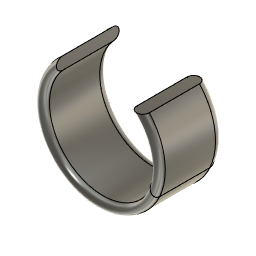
Correa (Autodesk Fusion 360 design; units mm, degrees)
Autodesk Fusion 360 part; units mm, degrees
sketch "Boceto1" plane through (0, 0, 0) normal (0, 0, 1) x (1, 0, 0)
  line L0 (0, 0) -> (30, 0)
  line L1 (30, 0) -> (30, 57)
  line L2 (30, 57) -> (0, 57)
  line L3 (0, 57) -> (0, 0)
  dimension "d1" = 57
  dimension "d2" = 30
  constraint horizontal L0
  constraint vertical L1
  constraint horizontal L2
  constraint vertical L3
  constraint coincident L0.start L3.end
  measures "d1" distance of L0.end L1.end
  measures "d2" distance of L1.end L2.end
extrude "Extruir1" add sketch "Boceto1" along normal blind 3 makes body 1
sketch "Boceto2" plane through (0, 0, 0) normal (0, 0, -1) x (1, 0, 0)
  line L0 (0, 0) -> (0, -57)
  line L1 (0, -57) -> (30, -57)
  line L2 (30, -57) -> (30, 0)
  line L3 (30, 0) -> (0, 0)
extrude "Extruir2" add sketch "Boceto2" against normal blind 10 thin wall 1 outside bodies 1
sketch "Boceto3" plane through (0, 58, 0) normal (0, 1, 0) x (-1, 0, 0)
  line L0 (-31, 0) -> (1, 0)
  line L1 (1, 0) -> (1, 10)
  line L2 (1, 10) -> (-31, 10)
  line L3 (-31, 10) -> (-31, 0)
  line L4 (-22.5, 6.5) -> (-7.5, 6.5)
  line L5 (-7.5, 6.5) -> (-7.5, 3.5)
  line L6 (-7.5, 3.5) -> (-22.5, 3.5)
  line L7 (-22.5, 3.5) -> (-22.5, 6.5)
  point P0 (-15, 3.5)
  point P1 (-15, 0)
  point P2 (-7.5, 5)
  point P3 (1, 5)
  dimension "d8" = 15
  dimension "d9" = 3
  constraint horizontal L4
  constraint vertical L5
  constraint horizontal L6
  constraint vertical L7
  constraint midpoint L6 P0
  constraint midpoint L0 P1
  constraint vertical P0 P1
  constraint midpoint L5 P2
  constraint midpoint L1 P3
  constraint horizontal P2 P3
  measures "d8" distance of L4.start L4.end
  measures "d9" distance of L4.end L5.end
extrude "Extruir3" cut sketch "Boceto3" against normal up to surface (1 mm away) contours L4 L5 L6 L7 bodies 1
sketch "Boceto4" plane through (0, 0, 3) normal (0, 0, 1) x (-1, 0, 0)
  line L0 (0, -57) -> (0, 0)
  line L1 (0, 0) -> (-30, 0)
  line L2 (-30, 0) -> (-30, -57)
  line L3 (-30, -57) -> (0, -57)
  line L4 (0, -28.5) -> (-30, -28.5)
  constraint midpoint L0 L4.start
  constraint midpoint L2 L4.end
ref_plane "PlanoDeObra1" through (0, 28.5, 0) normal (0, 1, 0) x (0, 0, 1)
sketch "Boceto5" plane through (0, 28.5, 0) normal (0, 1, 0) x (1, 0, 0)
  line L0 (-1, 0) -> (31, 0) construction
  line L1 (31, 0) -> (31, -10) construction
  line L2 (31, -10) -> (-1, -10) construction
  line L3 (-1, -10) -> (-1, 0) construction
  circle A0 centre (8, 9) radius 1
  arc A1 (36.536, 19.5388) -> (-1, -5) centre (15.0109, 11.4868) ccw
  arc A2 (31, -5) -> (36.536, 19.5388) centre (15.0346, 11.4957) ccw
  constraint tangent A1 A2
  constraint midpoint L1 A2.start
  constraint midpoint L3 A1.end
sketch "Boceto6" plane through (-1, 0, 0) normal (-1, 0, 0) x (0, -1, 0)
  line L0 (-58, 0) -> (1, 0)
  line L1 (1, 0) -> (1, 10)
  line L2 (1, 10) -> (-58, 10)
  line L3 (-58, 10) -> (-58, 0)
  line L4 (-38.5, 2.5) -> (-18.5, 2.5)
  arc A0 (-18.5, 2.5) -> (-18.5, 7.5) centre (-18.5, 5) ccw
  line L5 (-18.5, 7.5) -> (-38.5, 7.5)
  arc A1 (-38.5, 7.5) -> (-38.5, 2.5) centre (-38.5, 5) ccw
  line L6 (-38.5, 5) -> (-18.5, 5) construction
  point P0 (-28.5, 5)
  point P1 (-28.5, 5)
  dimension "d13" = 2.5
  dimension "d14" = 20
  constraint tangent L4 A0
  constraint tangent A0 L5
  constraint parallel L4 L5
  constraint tangent L5 A1
  constraint tangent L4 A1
  constraint horizontal L6
  constraint midpoint L6 P1
  constraint horizontal P1 P0
  constraint coincident P1 P0
  measures "d13" radius of A0
  measures "d14" distance of A0.end L5.end
sweep "Barrido1" add profiles "Boceto6" path "Boceto5" along A2 A1 section 1 contours L4 A0 L5 A1 separate body makes body 2
hidden bodies 1
